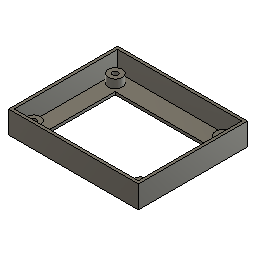
N-BLOCKS-FRAME-ASM (Autodesk Fusion 360 archive; units mm, degrees)
design "NBLOCKS-FRAME"
Autodesk Fusion 360 part; units mm, degrees
sketch "Sketch1" plane through (0, 0, 0) normal (0, 1, 0) x (1, 0, 0)
  line L0 (19.1, 14.575) -> (-19.1, 14.575) construction
  line L1 (-19.1, 14.575) -> (-19.1, -14.575) construction
  line L2 (-19.1, -14.575) -> (19.1, -14.575) construction
  line L3 (19.1, -14.575) -> (19.1, 14.575) construction
  line L4 (19.1, 14.575) -> (-19.1, -14.575) construction
  line L5 (-19.1, 14.575) -> (19.1, -14.575) construction
  circle A0 centre (-19.1, 14.575) radius 1
  circle A1 centre (19.1, 14.575) radius 1
  circle A2 centre (-19.1, -14.575) radius 1
  circle A3 centre (19.1, -14.575) radius 1
  circle A4 centre (-19.1, 14.575) radius 2.5
  circle A5 centre (19.1, 14.575) radius 2.5
  circle A6 centre (-19.1, -14.575) radius 2.5
  circle A7 centre (19.1, -14.575) radius 2.5
  line L6 (22.1, -18.4) -> (-22.1, -18.4)
  line L7 (-22.1, -18.4) -> (-22.1, 18.4)
  line L8 (-22.1, 18.4) -> (22.1, 18.4)
  line L9 (22.1, 18.4) -> (22.1, -18.4)
  line L10 (22.1, -18.4) -> (-22.1, 18.4) construction
  line L11 (-22.1, -18.4) -> (22.1, 18.4) construction
  line L12 (23.1, 19.4) -> (-23.1, 19.4)
  line L13 (-23.1, 19.4) -> (-23.1, -19.4)
  line L14 (-23.1, -19.4) -> (23.1, -19.4)
  line L15 (23.1, -19.4) -> (23.1, 19.4)
  line L16 (23.1, 19.4) -> (-23.1, -19.4) construction
  line L17 (-23.1, 19.4) -> (23.1, -19.4) construction
  line L18 (-16.5064, 18.4) -> (16.5064, 18.4)
  line L19 (16.5064, 18.4) -> (16.5064, -18.4)
  line L20 (16.5064, -18.4) -> (-16.5064, -18.4)
  line L21 (-16.5064, -18.4) -> (-16.5064, 18.4)
  line L22 (-16.5064, 18.4) -> (16.5064, -18.4) construction
  line L23 (16.5064, 18.4) -> (-16.5064, -18.4) construction
  line L24 (22.1, 11.9339) -> (-22.1, 11.9339)
  line L25 (-22.1, 11.9339) -> (-22.1, -11.9339)
  line L26 (-22.1, -11.9339) -> (22.1, -11.9339)
  line L27 (22.1, -11.9339) -> (22.1, 11.9339)
  line L28 (22.1, 11.9339) -> (-22.1, -11.9339) construction
  line L29 (-22.1, 11.9339) -> (22.1, -11.9339) construction
  dimension "d1" = 29.15
  dimension "d2" = 38.2
  dimension "d3" = 2
  dimension "d4" = 2
  dimension "d5" = 2
  dimension "d6" = 2
  dimension "d7" = 5
  dimension "d8" = 5
  dimension "d9" = 5
  dimension "d10" = 5
  dimension "d11" = 36.8
  dimension "d12" = 1
  dimension "d13" = 1
  dimension "d14" = 44.2
  constraint perpendicular L0 L1
  constraint parallel L0 L2
  constraint parallel L1 L3
  constraint horizontal L0
  constraint coincident L4 origin
  constraint coincident L5 origin
  constraint coincident L0.end L1.start
  constraint coincident L0.start L3.end
  constraint coincident L1.end L2.start
  constraint coincident L2.end L3.start
  constraint concentric A0 A4
  constraint concentric A1 A5
  constraint concentric A2 A6
  constraint concentric A3 A7
  constraint perpendicular L6 L7
  constraint parallel L6 L8
  constraint parallel L7 L9
  constraint horizontal L6
  constraint coincident L10 origin
  constraint coincident L11 origin
  constraint perpendicular L12 L13
  constraint parallel L12 L14
  constraint parallel L13 L15
  constraint horizontal L12
  constraint coincident L16 origin
  constraint coincident L17 origin
  constraint perpendicular L18 L19
  constraint parallel L18 L20
  constraint parallel L19 L21
  constraint horizontal L18
  constraint coincident L8 L18.start
  constraint coincident L22 origin
  constraint coincident L23 origin
  constraint perpendicular L24 L25
  constraint parallel L24 L26
  constraint parallel L25 L27
  constraint horizontal L24
  constraint coincident L9 L24.start
  constraint coincident L28 origin
  constraint coincident L29 origin
  measures "d1" distance of L0.end L1.end
  measures "d2" distance of L1.end L2.end
  measures "d3" diameter of A0
  measures "d4" diameter of A1
  measures "d5" diameter of A2
  measures "d6" diameter of A3
  measures "d7" diameter of A4
  measures "d8" diameter of A5
  measures "d9" diameter of A6
  measures "d10" diameter of A7
  measures "d11" distance of L6.end L7.end L0.start
  measures "d12" distance of L8 L12
  measures "d13" distance of L9 L15
  measures "d14" distance of L6.start L6.end L0.start
extrude "Extrude1" add sketch "Sketch1" along normal blind 8 contours L12 L13 L14 L15 makes body 1
extrude "Extrude2" add sketch "Sketch1" along normal blind 4 separate body contours A4 | A5 | A6 | A7 makes body 2 at (21.5969, 2.6667, -14.4504) makes body 3 at (-16.6031, 2.6667, 14.6996) makes body 4 at (-16.6031, 2.6667, -14.4504) makes body 5 at (21.5969, 2.6667, 14.6996)
extrude "Extrude3" add sketch "Sketch1" along normal blind 1 contours L6 L9 L19 L26 | L6 L19 L20 L21 L26 | L9 L19 L24 L26 L27 | L6 L7 L21 L26 | L8 L9 L19 L24 | L7 L21 L24 L25 L26 | L8 L18 L19 L21 L24 | L7 L8 L21 L24 bodies 1 2 3 4 5
